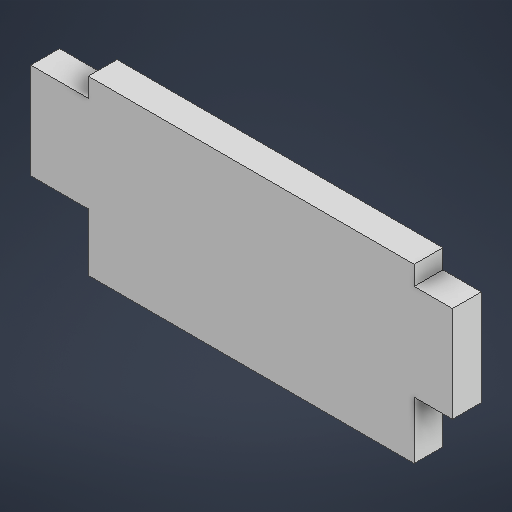
# Autodesk Inventor part: Frontrail
Saved by Autodesk Inventor 2027 (Build 310192000, 192)
## iProperties
Created: 2026-05-13
Part Number: Frontrail
Material: Generic
Document SubType Name: Modeling
Designer: alexy
Density: 1 g/cm^3
Appearance: Default
Author: alexy
Autodesk Inventor part; units mm, degrees
ref_plane "YZ Plane" through (0, 0, 0) normal (1, 0, 0) x (0, 1, 0)
ref_plane "XZ Plane" through (0, 0, 0) normal (0, 1, 0) x (-1, 0, 0)
ref_plane "XY Plane" through (0, 0, 0) normal (0, 0, 1) x (1, 0, 0)
sketch "Sketch1" plane through (0, 0, 0) normal (0, 0, 1) x (1, 0, 0)
  line L0 (0, 0) -> (34, 0)
  line L1 (34, 0) -> (34, 18)
  line L2 (34, 18) -> (0, 18)
  line L3 (0, 18) -> (0, 0)
  line L4 (-6, 16) -> (0, 16)
  line L5 (0, 16) -> (0, 6)
  line L6 (0, 6) -> (-6, 6)
  line L7 (-6, 6) -> (-6, 16)
  line L8 (-6, 16) -> (0, 6) construction
  line L9 (0, 16) -> (-6, 6) construction
  line L10 (38, 16) -> (34, 16)
  line L11 (34, 16) -> (34, 6)
  line L12 (34, 6) -> (38, 6)
  line L13 (38, 6) -> (38, 16)
  line L14 (38, 16) -> (34, 6) construction
  line L15 (34, 16) -> (38, 6) construction
  point P0 (-3, 11)
  point P1 (36, 11)
  point P2 (0, 16)
  dimension "d0" = 34
  dimension "d2" = 4
  dimension "d3" = 6
  dimension "d4" = 10
  dimension "d5" = 10
  dimension "d8" = 6
  dimension "d9" = 2
  constraints: 32 end point, 6 parallel, 4 midpoint, 3 horizontal, 3 perpendicular, 2 point on line, 1 horizontal alignment
  measures "d0" distance of L1.end L2.end
  measures "d2" distance of L10.start L10.end
  measures "d3" distance of L4.start L4.end
  measures "d4" distance of L6.end L4.start
  measures "d5" distance of L12.end L10.start
  measures "d8" distance of L0.start L5.end
  measures "d9" distance of L4.end L2.end
extrude "Extrusion1" add sketch "Sketch1" along normal blind 3
body "Solid1"
